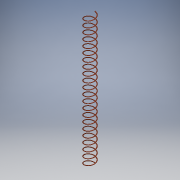
# Autodesk Inventor part: Ground_Antenna230mm_Helix
Saved by Autodesk Inventor 2018 (Build 220112000, 112)
## iProperties
Created: 2018-09-26
Part Number: Ground_Antenna230mm_Helix
Material: Copper
Document SubType Name: Modeling
Designer: Bradley
Density: 8.94 g/cm^3
Appearance: Copper - Satin
Author: Bradley
Autodesk Inventor part; units mm, degrees
ref_plane "YZ Plane" through (0, 0, 0) normal (1, 0, 0) x (0, 1, 0)
ref_plane "XZ Plane" through (0, 0, 0) normal (0, 1, 0) x (-1, 0, 0)
ref_plane "XY Plane" through (0, 0, 0) normal (0, 0, 1) x (1, 0, 0)
sketch "Sketch1" plane through (0, 0, 0) normal (1, 0, 0) x (0, 1, 0)
  circle A0 centre (45.575, 0) radius 3.175
  circle A1 centre (45.575, 0) radius 2.413
  line L0 (0, 0) -> (42.4, 0) construction
  line L1 (0, 0) -> (0, 54.3)
  dimension "d0" = 6.35
  dimension "d1" = 4.826
  dimension "d2" = 84.8
  dimension "d3" = 54.3
  constraints: 4 end point, 1 centre point, 1 coincident, 1 horizontal, 1 horizontal alignment, 1 point on line, 1 vertical, 2 other
  measures "d1" diameter of A1
  measures "d2" diameter of L0.end L1
  measures "d3" distance of L0.start L1.end
coil "Coil1" sketch "Sketch1" operation add axis through (0, 0, 0) along (0, 0, 1) pitch 54.3 turns 22 hand right
equation "\"d4\" = d3"
body "Solid1"
